fan-mounter v1 (Autodesk Fusion 360 design; units mm, degrees)
Autodesk Fusion 360 part; units mm, degrees
note: some values were not read from the file. Chosen so that the rebuilt part matches the saved one: which face or edge a step refers to; which pieces of a blend or face edit are solid. Set by a fixed rule: which sketch regions a step uses.
sketch "スケッチ1" plane through (0, 0, 0) normal (0, 0, 1) x (1, 0, 0)
  circle A0 centre (0, 0) radius 3
  circle A1 centre (0, 0) radius 3.9
  circle A2 centre (-11, 0) radius 0.9
  circle A3 centre (11, 0) radius 0.9
  line L0 (-12.5, 1.8) -> (12.5, 1.8)
  line L1 (12.5, -1.8) -> (-12.5, -1.8)
  line L2 (-12.5, 1.8) -> (-12.5, -1.8)
  line L3 (12.5, -1.8) -> (12.5, 1.8)
  line L4 (-12.5, 0) -> (12.5, 0)
  line L5 (0, 1.8) -> (0, -1.8)
  dimension "d3" = 6
  dimension "d4" = 7.8
  dimension "d5" = 1.8
  dimension "d8" = 3.6
  dimension "d16" = 25
  dimension "d17" = 1.5
  measures "d3" diameter of A0
  measures "d4" diameter of A1
  measures "d5" diameter of A2
  measures "d8" distance of L0.start L1.end
  measures "d16" distance of L1.start L1.end
  measures "d17" distance of A2.centre L2
extrude "押し出し1" add sketch "スケッチ1" along normal blind 1 contours A1 A3 L1 L3 L4 | A1 A3 L0 L3 L4 | A1 A2 L0 L2 L4 | A1 A2 L1 L2 L4 makes body 1 at (-8.877, -1.4793, 1) makes body 2 at (8.877, -1.4793, 1)
extrude "押し出し2" add sketch "スケッチ1" along normal blind 3 from surface at -1 contours A0 A1 L1 L4 | A0 A1 L0 L4 | A0 A1 L0 | A0 A1 L1 | A0 A1 L0 L4 | A0 A1 L1 L4 bodies 1 2
fillet "フィレット1" radius 0.8 10 edges at (-3.4598, -1.8, 0.5) (3.4598, -1.8, 0.5) (3.7883, -0.9265, 0) (3.7883, 0.9265, 0) (3.4598, 1.8, 0.5) (3.7883, 0.9265, 1) (3.7883, -0.9265, 1) (-3.9, 0, 1) (-3.4598, 1.8, 0.5) (-3.9, 0, 0) on bodies 1
